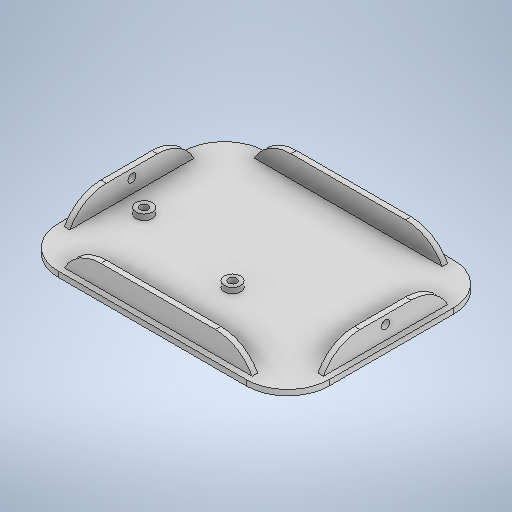
# Autodesk Inventor part: reduced_tortoise_2_base
Saved by Autodesk Inventor 2025.1 (Build 291241000, 241)
## iProperties
Created: 2025-04-14
Part Number: reduced_tortoise_2_base
Material: Generic
Document SubType Name: Modeling
Designer: Ian Ching
Density: 1 g/cm^3
Appearance: Default
Author: Ian Ching
Autodesk Inventor part; units mm, degrees
ref_plane "YZ Plane" through (0, 0, 0) normal (1, 0, 0) x (0, 1, 0)
ref_plane "XZ Plane" through (0, 0, 0) normal (0, 1, 0) x (-1, 0, 0)
ref_plane "XY Plane" through (0, 0, 0) normal (0, 0, 1) x (1, 0, 0)
sketch "Sketch5" plane through (0, 0, 0) normal (0, 1, 0) x (-1, 0, 0)
  line L0 (0, 0) -> (98, 0)
  line L1 (98, 0) -> (98, -75)
  line L2 (98, -75) -> (0, -75)
  line L3 (0, -75) -> (0, 0)
  dimension "d21" = 98
  dimension "d22" = 75
  constraints: 8 end point, 2 parallel, 1 horizontal, 1 perpendicular
  measures "d21" distance of L1.end L2.end
  measures "d22" distance of L0.end L1.end
extrude "Extrusion5" add sketch "Sketch5" along normal blind 2
fillet "Fillet3" radius 15 4 edges at (-98, 1, 0) (0, 1, 0) (0, 1, -75) (-98, 1, -75)
sketch "Sketch6" plane through (0, 2, 0) normal (0, 1, 0) x (1, 0, 0)
  line L0 (0, 60) -> (-2.1, 60)
  line L1 (-2.1, 60) -> (-2.1, 15)
  line L2 (-2.1, 15) -> (0, 15)
  line L3 (0, 15) -> (0, 60)
  line L4 (-95.9, 60) -> (-98, 60)
  line L5 (-98, 60) -> (-98, 15)
  line L6 (-98, 15) -> (-95.9, 15)
  line L7 (-95.9, 15) -> (-95.9, 60)
  line L8 (0, 15) -> (0, 60) projected
  line L9 (-98, 60) -> (-98, 15) projected
  line L10 (-95.9, 60) -> (-93.9, 60)
  line L11 (-93.9, 60) -> (-93.9, 15)
  line L12 (-93.9, 15) -> (-95.9, 15)
  line L13 (-95.9, 15) -> (-95.9, 60)
  line L14 (-4.1, 60) -> (-2.1, 60)
  line L15 (-2.1, 60) -> (-2.1, 15)
  line L16 (-2.1, 15) -> (-4.1, 15)
  line L17 (-4.1, 15) -> (-4.1, 60)
  line L18 (-15, 75) -> (-83, 75) projected
  line L19 (-83, 75) -> (-15, 75)
  line L20 (-15, 75) -> (-15, 72.9)
  line L21 (-15, 72.9) -> (-83, 72.9)
  line L22 (-83, 72.9) -> (-83, 75)
  arc A0 (-98, 15) -> (-83, 0) centre (-83, 15) ccw projected
  line L23 (-83, 0) -> (-15, 0)
  line L24 (-15, 0) -> (-15, 2.1)
  line L25 (-15, 2.1) -> (-83, 2.1)
  line L26 (-83, 2.1) -> (-83, 0)
  line L27 (-83, 72.9) -> (-15, 72.9)
  line L28 (-15, 72.9) -> (-15, 70.9)
  line L29 (-15, 70.9) -> (-83, 70.9)
  line L30 (-83, 70.9) -> (-83, 72.9)
  line L31 (-83, 2.1) -> (-15, 2.1)
  line L32 (-15, 2.1) -> (-15, 4.1)
  line L33 (-15, 4.1) -> (-83, 4.1)
  line L34 (-83, 4.1) -> (-83, 2.1)
  point P0 (0, 0)
  point P1 (0, 37.5)
  point P2 (-98, 37.5)
  point P3 (-95.9, 37.5)
  point P4 (-2.1, 37.5)
  point P5 (-2.1, 60)
  dimension "d26" = 2.1
  dimension "d27" = 45
  dimension "d28" = 2.1
  dimension "d29" = 45
  dimension "d30" = 2
  dimension "d31" = 45
  dimension "d32" = 2
  dimension "d33" = 45
  dimension "d57" = 68
  dimension "d58" = 2.1
  dimension "d59" = 68
  dimension "d60" = 2.1
  dimension "d61" = 68
  dimension "d62" = 2
  dimension "d63" = 68
  dimension "d64" = 2
  constraints: 64 end point, 16 parallel, 8 horizontal, 8 midpoint, 8 perpendicular
  measures "d26" distance of L2.end L1.end
  measures "d27" distance of L1.end L0.end
  measures "d28" distance of L6.end L5.end
  measures "d29" distance of L5.end L4.end
  measures "d30" distance of L11.end L12.end
  measures "d31" distance of L10.end L11.end
  measures "d32" distance of L15.end L16.end
  measures "d33" distance of L14.end L15.end
  measures "d57" distance of L20.end L21.end
  measures "d58" distance of L19.end L20.end
  measures "d59" distance of L25.end L24.end
  measures "d60" distance of L24.end L23.end
  measures "d61" distance of L28.end L29.end
  measures "d62" distance of L27.end L28.end
  measures "d63" distance of L33.end L32.end
  measures "d64" distance of L32.end L31.end
extrude "Extrusion6" add sketch "Sketch6" along normal blind 8 contours L1 L16 L17 L14 | L10 L11 L12 L7 | L28 L29 L30 L21 | L34 L33 L32 L25
sketch "Sketch7" plane through (-2.1, 2, -15) normal (1, 0, 0) x (0, 0, -1)
  line L0 (0, 0) -> (45, 0) projected
  line L1 (0, 0) -> (45, 0)
  line L2 (45, 0) -> (45, 5)
  line L3 (45, 5) -> (0, 5)
  line L4 (0, 5) -> (0, 0)
  circle A0 centre (22.5, 5) radius 1.5
  point P0 (-15, -2)
  dimension "d36" = 45
  dimension "d37" = 5
  dimension "d38" = 3
  constraints: 8 end point, 2 parallel, 1 centre point, 1 horizontal, 1 midpoint, 1 perpendicular
  measures "d36" distance of L3.end L2.end
  measures "d37" distance of L2.end L1.end
  measures "d38" diameter of A0
extrude "Extrusion7" cut sketch "Sketch7" against normal blind 100 contours A0 L3 | L3 A0
fillet "Fillet4" radius 15 4 edges at (-3.1, 10, -15) (-3.1, 10, -60) (-94.9, 10, -60) (-94.9, 10, -15)
sketch "Sketch8" plane through (0, 2, 0) normal (0, 1, 0) x (1, 0, 0)
  line L0 (-88, 18.5) -> (-34, 18.5)
  line L1 (-34, 18.5) -> (-34, 56.5)
  line L2 (-34, 56.5) -> (-88, 56.5)
  line L3 (-88, 56.5) -> (-88, 18.5)
  line L4 (-34, 18.5) -> (-46.5, 18.5)
  line L5 (-46.5, 18.5) -> (-46.5, 26.5)
  line L6 (-46.5, 26.5) -> (-34, 26.5)
  line L7 (-34, 26.5) -> (-34, 18.5)
  line L8 (-88, 18.5) -> (-85.5, 18.5)
  line L9 (-85.5, 18.5) -> (-85.5, 33.5)
  line L10 (-85.5, 33.5) -> (-88, 33.5)
  line L11 (-88, 33.5) -> (-88, 18.5)
  circle A0 centre (-85.5, 33.5) radius 3
  circle A1 centre (-46.5, 26.5) radius 3
  line L12 (-98, 60) -> (-98, 15) projected
  line L13 (-98, 37.5) -> (0, 37.5)
  line L14 (0, 15) -> (0, 60) projected
  line L15 (-98, 37.5) -> (-88, 37.5)
  point P0 (0, 0)
  dimension "d42" = 54
  dimension "d43" = 38
  dimension "d44" = 12.5
  dimension "d45" = 8
  dimension "d46" = 2.5
  dimension "d47" = 15
  dimension "d48" = 6
  dimension "d49" = 6
  dimension "d50" = 10
  constraints: 28 end point, 6 parallel, 3 horizontal, 3 midpoint, 3 perpendicular, 2 centre point, 2 coincident, 1 point on line
  measures "d42" distance of L2.end L1.end
  measures "d43" distance of L1.end L0.end
  measures "d44" distance of L5.end L6.end
  measures "d45" distance of L4.end L5.end
  measures "d46" distance of L10.end L9.end
  measures "d47" distance of L9.end L8.end
  measures "d48" diameter of A0
  measures "d49" diameter of A1
  measures "d50" distance of L15.end L13.start
extrude "Extrusion8" add sketch "Sketch8" along normal blind 2 contours A0 L3 | L3 L10 L9 A0 | L9 L10 L3 A0 | A1 L6 L5 | L5 L6 A1
sketch "Sketch9" plane through (-85.5, 4, -33.5) normal (0, 1, 0) x (1, 0, 0)
  circle A0 centre (0, 0) radius 3 projected
  circle A1 centre (0, 0) radius 1.5
  circle A2 centre (39, -7) radius 3 projected
  circle A3 centre (39, -7) radius 1.5
  point P0 (85.5, -33.5)
  dimension "d53" = 3
  dimension "d54" = 3
  constraints: 2 centre point, 2 coincident
  measures "d53" diameter of A1
  measures "d54" diameter of A3
extrude "Extrusion9" cut sketch "Sketch9" against normal blind 3 contours A1 | A3
fillet "Fillet5" radius 15 4 edges at (-83, 10, -3.1) (-15, 10, -3.1) (-15, 10, -71.9) (-83, 10, -71.9)
body "Solid2"
